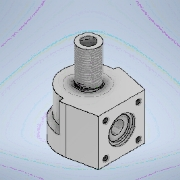
# Autodesk Inventor part: 00.32.001 "Housing "
Saved by Autodesk Inventor 2025.2 (Build 292293000, 293)
## iProperties
Created: 2024-12-20
Part Number: 00.32.001 "Housing "
Material: Steel
Document SubType Name: Modeling
Designer: Anna
Language: en-US
Size Designation: Корпус 00.32(різьба)
Categories: <MemberInstance><Categories><Category DisplayName="Other Parts" InternalName="5aa15e00-363f-49f2-933f-16f664388e3f" Mnemonic="OTHER"/><Category DisplayName="DataType" InternalName="23b78d0f-2648-40c6-8793-ca6db495c9e8" Mnemonic="DATATYPE"><CategoryParameter DisplayName="DisplayName" InternalName="05415f3d-3907-474b-a020-eb9d644f4cf3" Mnemonic="DISPLAYNAME"/><CategoryParameter DisplayName="Standard" InternalName="0c0a119c-1e12-4c84-803f-101930972f5e" Mnemonic="STANDARD"/><CategoryParameter DisplayName="Description" InternalName="13903e3d-64b1-4950-80da-f627842ea37f" Mnemonic="DESCRIPTION"/><CategoryParameter DisplayName="Designation" InternalName="2675968c-4ce5-49e0-a4f5-552d29089031" Mnemonic="DESIGNATION"/><CategoryParameter DisplayName="Default Row" InternalName="2af9ec52-faaa-4026-b378-f9fa4afca842" Mnemonic="DEFAULTROW"/><CategoryParameter DisplayName="Folder Name" InternalName="3f06958e-8713-4116-9be7-ed6184ecc97b" Mnemonic="FOLDERNAME"/><CategoryParameter DisplayName="Revision Guid" InternalName="45a75005-10b1-4dfc-8d6d-dfe629f0b93c" Mnemonic="REVISIONGUID"/><CategoryParameter DisplayName="FileName" InternalName="8b46a4cc-9585-4fed-90c3-899f57e09a73" Mnemonic="FILENAME"/><CategoryParameter DisplayName="StdsOrg" InternalName="8f5914e1-4693-403f-8ab5-d37768198c9d" Mnemonic="STDSORG"/><CategoryParameter DisplayName="Family Version" InternalName="914462f6-6e19-4b14-ba84-155b9680b1d0" Mnemonic="FAMILYREVISION"/><CategoryParameter DisplayName="Standard Revision" InternalName="91d5a463-65c2-4fde-b823-3b7fea5e8e17" Mnemonic="STANDARDREVISION"/><CategoryParameter DisplayName="Member Revision" InternalName="a65d44b9-392f-4f4f-857b-e4b3d54996fe" Mnemonic="MEMBERREVISION"/><CategoryParameter DisplayName="ClipFormat" InternalName="bc51e27b-3422-4e78-93ef-cec197ddf230" Mnemonic="CLIPFORMAT"/><CategoryParameter DisplayName="Manufacturer" InternalName="cd6c7a72-a28a-4e50-99a9-2c7f4e13e5ad" Mnemonic="MANUFACTURER"/><CategoryParameter DisplayName="InternalName" InternalName="cf1d0246-76d9-4b4a-8305-fa0409afb5c1" Mnemonic="INTERNALNAME"/><CategoryParameter DisplayName="IsMetric" InternalName="e2385c5b-1ea4-4823-96a8-8de651266ec3" Mnemonic="ISMETRIC"/><Category DisplayName="Part" InternalName="c0e0b642-3bcb-4cc8-9e80-f96d35c4afa4" Mnemonic="PART"><CategoryParameter DisplayName="Part Number" InternalName="016b6077-bfbe-49bd-92c9-d8d59c39c941" Mnemonic="PARTNUMBER"/><CategoryParameter DisplayName="Stock Number" InternalName="4dba7c1c-e26c-444e-836c-b08b433409a8" Mnemonic="STOCKNUMBER"/><CategoryParameter DisplayName="Material Key" InternalName="5c9a8adb-dd2b-4535-b97f-0a94a95fe41f" Mnemonic="MATERIALKEY"/><CategoryParameter DisplayName="Material" InternalName="818a152a-d3c3-49ca-80ee-df7d91421b8e" Mnemonic="MATERIAL"/></Category></Category></Categories><FamilyTemplate Id="00.32.001 Корпус"><FamilyTemplateParameters><FamilyTemplateParameter ObjectType="kPartComponentDefinitionObject" ValueType="xs:string" Id="3" SubObjectId="Material"/><FamilyTemplateParameter ObjectType="kPropertyObject" ValueType="xs:string" Id="36" ObjectReferenceKey="{32853F0F-3444-11d1-9E93-0060B03C1CA6}" SubObjectId="5"/><FamilyTemplateParameter ObjectType="kPropertyObject" ValueType="xs:string" Id="37" ObjectReferenceKey="{32853F0F-3444-11d1-9E93-0060B03C1CA6}" SubObjectId="52"/></FamilyTemplateParameters></FamilyTemplate><CategoryParameterMap><ParamToTemplateMap><ParamToTemplate CategoryParameter="//CategoryParameter[@InternalName='cf1d0246-76d9-4b4a-8305-fa0409afb5c1']" ConstantValue="bf1ea542-7cda-4015-a09c-42ca0947e2f3"/><ParamToTemplate CategoryParameter="//CategoryParameter[@InternalName='45a75005-10b1-4dfc-8d6d-dfe629f0b93c']" ConstantValue="73068be6-1193-4558-8ae4-9fc5fdbda4b4"/><ParamToTemplate CategoryParameter="//CategoryParameter[@InternalName='3f06958e-8713-4116-9be7-ed6184ecc97b']" ConstantValue="00.32.001 Корпус"/><ParamToTemplate CategoryParameter="//CategoryParameter[@InternalName='8f5914e1-4693-403f-8ab5-d37768198c9d']" TemplateParameter="8"/><ParamToTemplate CategoryParameter="//CategoryParameter[@InternalName='0c0a119c-1e12-4c84-803f-101930972f5e']" TemplateParameter="9"/><ParamToTemplate CategoryParameter="//CategoryParameter[@InternalName='91d5a463-65c2-4fde-b823-3b7fea5e8e17']" TemplateParameter="10"/><ParamToTemplate CategoryParameter="//CategoryParameter[@InternalName='cd6c7a72-a28a-4e50-99a9-2c7f4e13e5ad']" TemplateParameter="11"/><ParamToTemplate CategoryParameter="//CategoryParameter[@InternalName='13903e3d-64b1-4950-80da-f627842ea37f']" TemplateParameter="12"/><ParamToTemplate CategoryParameter="//CategoryParameter[@InternalName='05415f3d-3907-474b-a020-eb9d644f4cf3']" ConstantValue="00.32.001 Корпус"/><ParamToTemplate CategoryParameter="//CategoryParameter[@InternalName='914462f6-6e19-4b14-ba84-155b9680b1d0']" ConstantValue="11"/><ParamToTemplate CategoryParameter="//CategoryParameter[@InternalName='bc51e27b-3422-4e78-93ef-cec197ddf230']" ConstantValue="CF_INVENTOR.STDPARTS"/><ParamToTemplate CategoryParameter="//CategoryParameter[@InternalName='e2385c5b-1ea4-4823-96a8-8de651266ec3']" ConstantValue="true"/><ParamToTemplate CategoryParameter="//CategoryParameter[@InternalName='2af9ec52-faaa-4026-b378-f9fa4afca842']" ConstantValue="1"/><ParamToTemplate CategoryParameter="//CategoryParameter[@InternalName='8b46a4cc-9585-4fed-90c3-899f57e09a73']" ConstantValue="Корпус 00.32-01"/><ParamToTemplate CategoryParameter="//CategoryParameter[@InternalName='a65d44b9-392f-4f4f-857b-e4b3d54996fe']" ConstantValue="d5eba91d-a7b9-454c-b222-4a6c4353da5b"/><ParamToTemplate CategoryParameter="//CategoryParameter[@InternalName='a65d44b9-392f-4f4f-857b-e4b3d54996fe']" ConstantValue="d5eba91d-a7b9-454c-b222-4a6c4353da5b"/><ParamToTemplate CategoryParameter="//CategoryParameter[@InternalName='2675968c-4ce5-49e0-a4f5-552d29089031']" TemplateParameter="37"/><ParamToTemplate CategoryParameter="//CategoryParameter[@InternalName='818a152a-d3c3-49ca-80ee-df7d91421b8e']" TemplateParameter="3"/><ParamToTemplate CategoryParameter="//CategoryParameter[@InternalName='016b6077-bfbe-49bd-92c9-d8d59c39c941']" TemplateParameter="36"/></ParamToTemplateMap></CategoryParameterMap></MemberInstance>
Mass: 1348.16 g
Surface Area: 1237.26 cm^2
Volume: 1348.16 cm^3
Density: 7.85 g/cm^3
Appearance: Aluminum - Polished
IsCustomPart: 1
Author: Anna
Autodesk Inventor part; units mm, degrees
ref_plane "YZ Plane" through (0, 0, 0) normal (1, 0, 0) x (0, 1, 0)
ref_plane "XZ Plane" through (0, 0, 0) normal (0, 1, 0) x (-1, 0, 0)
ref_plane "XY Plane" through (0, 0, 0) normal (0, 0, 1) x (1, 0, 0)
sketch "Sketch19" plane through (0, 0, 0) normal (0, 1, 0) x (-1, 0, 0)
  arc A0 (-13.4483, -63.5936) -> (-13.4483, 63.5936) centre (0, 0) ccw
  line L0 (-73, -51) -> (-73, 51)
  line L1 (-73, 51) -> (-13.4483, 63.5936)
  line L2 (-73, -51) -> (-13.4483, -63.5936)
  dimension "d91" = 130
  dimension "d93" = 102
  constraints: 6 end point, 2 point on circle, 2 tangent, 1 centre point, 1 coincident, 1 vertical
  measures "d91" diameter of A0
  measures "d93" distance of L0.start L0.end
extrude "Extrusion18" add sketch "Sketch19" along normal blind 37
sketch "Sketch20" plane through (0, 37, 0) normal (0, 1, 0) x (1, 0, 0)
  arc A0 (0, 56) -> (0, -56) centre (0, 0) ccw
  line L0 (0, -56) -> (0, -65)
  line L1 (0, 56) -> (0, 65)
  arc A1 (13.4483, 63.5936) -> (13.4483, -63.5936) centre (0, 0) ccw projected
  line L2 (13.4483, -63.5936) -> (73, -51) projected
  line L3 (73, -51) -> (73, 51) projected
  line L4 (73, 51) -> (13.4483, 63.5936) projected
  dimension "d96" = 112
  constraints: 4 end point, 3 point on circle, 2 vertical, 1 centre point, 1 coincident
  measures "d96" diameter of A0
extrude "Extrusion19" add sketch "Sketch20" along normal blind 65 contours L1 A1 L4 L3 L2 L0 A0
chamfer "Chamfer2" distance 9 angle 45 1 edges at (-56, 37, 0)
sketch "Sketch21" plane through (0, 0, 0) normal (0, -1, 0) x (1, 0, 0)
  circle A0 centre (0, 0) radius 29
  dimension "d102" = 58
  constraints: 1 centre point, 1 coincident
  measures "d102" diameter of A0
extrude "Extrusion20" cut sketch "Sketch21" against normal blind 4
sketch "Sketch22" plane through (0, 4, 0) normal (0, -1, 0) x (1, 0, 0)
  circle A0 centre (0, 0) radius 24
  dimension "d105" = 48
  constraints: 1 centre point, 1 coincident
  measures "d105" diameter of A0
extrude "Extrusion21" cut sketch "Sketch22" against normal blind 19
sketch "Sketch23" plane through (0, 0, 0) normal (0, -1, 0) x (1, 0, 0)
  circle A0 centre (-54, 0) radius 5
  circle A1 centre (54, 0) radius 5
  point P0 (0, 0)
  dimension "d109" = 10
  dimension "d110" = 10
  constraints: 2 centre point
  measures "d109" diameter of A0
  measures "d110" diameter of A1
extrude "Extrusion22" cut sketch "Sketch23" against normal blind 12
sketch "Sketch24" plane through (73, 0, 51) normal (1, 0, 0) x (0, 0, -1)
  line L0 (0, 102) -> (102, 102) projected
  line L1 (102, 0) -> (102, 102) projected
  line L2 (0, 0) -> (0, 102) projected
  line L3 (0, 0) -> (102, 0) projected
  circle A0 centre (51, 51) radius 29
  point P0 (51, 0)
  dimension "d113" = 58
  constraints: 1 centre point
  measures "d113" diameter of A0
extrude "Extrusion23" cut sketch "Sketch24" against normal blind 5 contours A0
sketch "Sketch25" plane through (68, 51, 0) normal (1, 0, 0) x (0, 0, -1)
  circle A0 centre (0, 0) radius 24
  point P0 (0, -51)
  dimension "d116" = 48
  constraints: 1 centre point
  measures "d116" diameter of A0
extrude "Extrusion24" cut sketch "Sketch25" against normal blind 4
sketch "Sketch26" plane through (64, 51, 0) normal (1, 0, 0) x (0, 0, -1)
  circle A0 centre (0, 0) radius 13.5
  point P0 (0, -51)
  dimension "d119" = 27
  constraints: 1 centre point
  measures "d119" diameter of A0
extrude "Extrusion25" cut sketch "Sketch26" against normal blind 38
sketch "Sketch27" plane through (73, 0, 51) normal (1, 0, 0) x (0, 0, -1)
  line L0 (15, 86) -> (87, 14) construction
  line L1 (87, 86) -> (15, 14) construction
  circle A0 centre (15, 86) radius 5
  circle A1 centre (87, 86) radius 5
  circle A2 centre (87, 14) radius 5
  circle A3 centre (15, 14) radius 5
  point P0 (51, 0)
  point P1 (51, 50)
  dimension "d125" = 72
  dimension "d126" = 72
  dimension "d127" = 10
  dimension "d128" = 10
  dimension "d129" = 10
  dimension "d130" = 10
  constraints: 4 centre point, 4 coincident, 4 end point, 2 midpoint
  measures "d125" distance of L0.end L1.end
  measures "d126" distance of L1.start L0.end
  measures "d127" diameter of A0
  measures "d128" diameter of A1
  measures "d129" diameter of A2
  measures "d130" diameter of A3
extrude "Extrusion26" cut sketch "Sketch27" against normal blind 16
sketch "Sketch28" plane through (0, 102, 0) normal (0, 1, 0) x (1, 0, 0)
  circle A0 centre (0, 0) radius 22.5
  dimension "d133" = 45
  constraints: 1 centre point, 1 coincident
  measures "d133" diameter of A0
extrude "Extrusion27" add sketch "Sketch28" along normal blind 81
sketch "Sketch29" plane through (0, 183, 0) normal (0, 1, 0) x (1, 0, 0)
  circle A0 centre (0, 0) radius 13.5
  dimension "d136" = 27
  constraints: 1 centre point, 1 coincident
  measures "d136" diameter of A0
extrude "Extrusion28" cut sketch "Sketch29" against normal blind 26
sketch "Sketch30" plane through (0, 157, 0) normal (0, 1, 0) x (1, 0, 0)
  circle A0 centre (0, 0) radius 8.5
  dimension "d139" = 17
  constraints: 1 centre point, 1 coincident
  measures "d139" diameter of A0
extrude "Extrusion29" cut sketch "Sketch30" against normal blind 91
sketch "Sketch31" plane through (0, 0, 0) normal (0, 0, 1) x (1, 0, 0)
  line L0 (22.5, 102) -> (22.5, 183) projected
  line L1 (22.5, 102) -> (22.5, 106)
  line L2 (22.5, 102) -> (26.5, 102) construction
  circle A0 centre (22.5, 104) radius 2
  line L3 (-92.6, 0) -> (100.6, 0) projected
  line L4 (0, -36.6) -> (0, 219.6) projected
  point P0 (0, 0)
  dimension "d142" = 4
  dimension "d143" = 90
  constraints: 4 end point, 1 centre point, 1 collinear, 1 horizontal, 1 midpoint, 1 perpendicular, 1 point on line
  measures "d142" distance of L1.start L1.end
  measures "d143" angle of L2 L1
revolve "Revolution1" cut sketch "Sketch31" angle 360 about axis through (0, -10, 0) along (0, 1, 0)
sketch "Sketch32" plane through (0, 23, 0) normal (0, -1, 0) x (1, 0, 0)
  circle A0 centre (0, 0) radius 29
  dimension "d146" = 58
  constraints: 1 centre point, 1 coincident
  measures "d146" diameter of A0
extrude "Extrusion30" cut sketch "Sketch32" against normal blind 43
thread "Thread10" size "M20x2.5" class "6H" standard "ANSI Metric M Profile" full length
thread "Thread11" size "M12x1.75" class "6H" standard "ANSI Metric M Profile" full length
thread "Thread12" size "M12x1.75" class "6H" standard "ANSI Metric M Profile" full length
thread "Thread13" size "M12x1.75" class "6H" standard "ANSI Metric M Profile" full length
thread "Thread14" size "M12x1.75" class "6H" standard "ANSI Metric M Profile" full length
thread "Thread15" size "M45x4.5" class "6g" standard "ANSI Metric M Profile" full length
thread "Thread16" size "M12x1.75" class "6H" standard "ANSI Metric M Profile" full length
thread "Thread17" size "M12x1.75" class "6H" standard "ANSI Metric M Profile" full length
body "Solid3"
